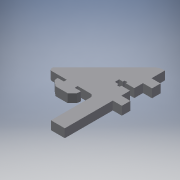
# Autodesk Inventor part: Y-Motor-Brace
Saved by Autodesk Inventor 2017 (Build 210142000, 142)
## iProperties
Created: 2016-07-21
Part Number: Y-Motor-Brace
Material: Generic
Document SubType Name: Modeling
Designer: User
Density: 1 g/cm^3
Appearance: Default
Author: User
Autodesk Inventor part; units mm, degrees
(part 1 of 2)
ref_plane "YZ Plane" through (0, 0, 0) normal (1, 0, 0) x (0, 1, 0)
ref_plane "XZ Plane" through (0, 0, 0) normal (0, 1, 0) x (-1, 0, 0)
ref_plane "XY Plane" through (0, 0, 0) normal (0, 0, 1) x (1, 0, 0)
sketch "Sketch1" plane through (0, 0, 0) normal (0, 0, 1) x (1, 0, 0)
  line L0 (977.8791, 108.9161) -> (977.8791, 115.0161)
  line L1 (977.8791, 115.0161) -> (984.2291, 115.0161)
  line L2 (984.2291, 115.0161) -> (984.2291, 121.0067)
  line L3 (984.2291, 121.0067) -> (977.8884, 121.0067)
  line L4 (977.8884, 121.0067) -> (977.8884, 130.4067)
  line L5 (977.8884, 130.4067) -> (977.2021, 130.4067)
  line L6 (977.2021, 130.4067) -> (976.6789, 130.3897)
  line L7 (976.6789, 130.3897) -> (976.1579, 130.3385)
  line L8 (976.1579, 130.3385) -> (975.6413, 130.2534)
  line L9 (975.6413, 130.2534) -> (975.1315, 130.1346)
  line L10 (975.1315, 130.1346) -> (974.6306, 129.9827)
  line L11 (974.6306, 129.9827) -> (974.1405, 129.7985)
  line L12 (974.1405, 129.7985) -> (973.6636, 129.5825)
  line L13 (973.6636, 129.5825) -> (973.2019, 129.3358)
  line L14 (973.2019, 129.3358) -> (972.7572, 129.0595)
  line L15 (972.7572, 129.0595) -> (972.3316, 128.7547)
  line L16 (972.3316, 128.7547) -> (971.9269, 128.4227)
  line L17 (971.9269, 128.4227) -> (971.5447, 128.0649)
  line L18 (971.5447, 128.0649) -> (937.996, 94.5327)
  line L19 (937.996, 94.5327) -> (938.0208, 94.542)
  line L20 (938.0208, 94.542) -> (937.2042, 93.7246)
  spline S0 degree 3 poles (937.2042, 93.7246) (937.0556, 93.5758) (936.9321, 93.4056) (936.8368, 93.2181) knots 21 21 21 21 22 22 22 22
  line L21 (937.2042, 93.7246) -> (937.0556, 93.5758) construction
  line L22 (937.0556, 93.5758) -> (936.9321, 93.4056) construction
  line L23 (936.9321, 93.4056) -> (936.8368, 93.2181) construction
  spline S1 degree 3 poles (936.8368, 93.2181) (936.7414, 93.0307) (936.6766, 92.8306) (936.6438, 92.6229) knots 22 22 22 22 23 23 23 23
  line L24 (936.8368, 93.2181) -> (936.7414, 93.0307) construction
  line L25 (936.7414, 93.0307) -> (936.6766, 92.8306) construction
  line L26 (936.6766, 92.8306) -> (936.6438, 92.6229) construction
  spline S2 degree 3 poles (936.6438, 92.6229) (936.611, 92.4151) (936.6112, 92.2048) (936.6443, 91.9971) (936.6774, 91.7895) (936.7425, 91.5895) (936.8381, 91.4022) knots 23 23 23 23 24 24 24 25 25 25 25
  line L27 (936.6438, 92.6229) -> (936.611, 92.4151) construction
  line L28 (936.611, 92.4151) -> (936.6112, 92.2048) construction
  line L29 (936.6112, 92.2048) -> (936.6443, 91.9971) construction
  line L30 (936.6443, 91.9971) -> (936.6774, 91.7895) construction
  line L31 (936.6774, 91.7895) -> (936.7425, 91.5895) construction
  line L32 (936.7425, 91.5895) -> (936.8381, 91.4022) construction
  spline S3 degree 3 poles (936.8381, 91.4022) (936.9337, 91.2148) (937.0574, 91.0448) (937.2062, 90.8962) knots 25 25 25 25 26 26 26 26
  line L33 (936.8381, 91.4022) -> (936.9337, 91.2148) construction
  line L34 (936.9337, 91.2148) -> (937.0574, 91.0448) construction
  line L35 (937.0574, 91.0448) -> (937.2062, 90.8962) construction
  spline S4 degree 3 poles (937.2062, 90.8962) (937.355, 90.7476) (937.5252, 90.6241) (937.7127, 90.5287) knots 26 26 26 26 27 27 27 27
  line L36 (937.2062, 90.8962) -> (937.355, 90.7476) construction
  line L37 (937.355, 90.7476) -> (937.5252, 90.6241) construction
  line L38 (937.5252, 90.6241) -> (937.7127, 90.5287) construction
  spline S5 degree 3 poles (937.7127, 90.5287) (937.9002, 90.4334) (938.1002, 90.3685) (938.3079, 90.3358) knots 27 27 27 27 28 28 28 28
  line L39 (937.7127, 90.5287) -> (937.9002, 90.4334) construction
  line L40 (937.9002, 90.4334) -> (938.1002, 90.3685) construction
  line L41 (938.1002, 90.3685) -> (938.3079, 90.3358) construction
  spline S6 degree 3 poles (938.3079, 90.3358) (938.411, 90.3195) (938.5151, 90.3114) (938.6195, 90.3114) knots 28 28 28 28 29 29 29 29
  line L42 (938.3079, 90.3358) -> (938.411, 90.3195) construction
  line L43 (938.411, 90.3195) -> (938.5151, 90.3114) construction
  line L44 (938.5151, 90.3114) -> (938.6195, 90.3114) construction
  line L45 (938.6195, 90.3114) -> (949.0602, 90.3114)
  line L46 (949.0602, 90.3114) -> (949.0602, 88.2628)
  line L47 (949.0602, 88.2628) -> (944.6963, 88.2628)
  line L48 (944.6963, 88.2628) -> (944.6963, 87.5628)
  line L49 (944.6963, 87.5628) -> (945.0555, 85.6914)
  line L50 (945.0555, 85.6914) -> (949.0203, 82.4161)
  line L51 (949.0203, 82.4161) -> (957.4678, 82.4161)
  line L52 (957.4678, 82.4161) -> (960.7553, 85.6883)
  line L53 (960.7553, 85.6883) -> (961.0631, 87.5612)
  line L54 (961.0631, 87.5612) -> (961.0631, 88.2612)
  line L55 (961.0631, 88.2612) -> (956.7022, 88.2612)
  line L56 (956.7022, 88.2612) -> (956.7022, 90.3082)
  line L57 (956.7022, 90.3082) -> (965.3221, 90.3082)
  line L58 (965.3221, 90.3082) -> (966.007, 90.2748)
  line L59 (966.007, 90.2748) -> (966.66, 90.0653)
  line L60 (966.66, 90.0653) -> (967.2366, 89.6939)
  line L61 (967.2366, 89.6939) -> (967.6973, 89.186)
  line L62 (967.6973, 89.186) -> (968.0109, 88.5761)
  line L63 (968.0109, 88.5761) -> (968.1559, 87.9058)
  line L64 (968.1559, 87.9058) -> (968.1559, 60.091)
  line L65 (968.1559, 60.091) -> (977.8791, 60.091)
  line L66 (977.8791, 60.091) -> (977.8791, 93.8161)
  line L67 (977.8791, 93.8161) -> (984.2291, 93.8161)
  line L68 (984.2291, 93.8161) -> (984.2291, 99.8161)
  line L69 (984.2291, 99.8161) -> (977.8791, 99.8161)
  line L70 (977.8791, 99.8161) -> (977.8791, 105.9161)
  line L71 (977.8791, 105.9161) -> (971.879, 105.9161)
  line L72 (971.879, 105.9161) -> (971.879, 104.6661)
  line L73 (971.879, 104.6661) -> (969.8791, 104.6661)
  line L74 (969.8791, 104.6661) -> (969.8791, 105.9161)
  line L75 (969.8791, 105.9161) -> (967.2291, 105.9161)
  line L76 (967.2291, 105.9161) -> (967.2291, 108.9161)
  line L77 (967.2291, 108.9161) -> (969.8791, 108.9161)
  line L78 (969.8791, 108.9161) -> (969.8791, 110.1661)
  line L79 (969.8791, 110.1661) -> (971.879, 110.1661)
  line L80 (971.879, 110.1661) -> (971.879, 108.9161)
  line L81 (971.879, 108.9161) -> (977.8791, 108.9161)
  line L82 (967.192, 195.3235) -> (966.942, 195.9235)
  line L83 (966.942, 195.9235) -> (966.542, 196.4485)
  line L84 (966.542, 196.4485) -> (966.017, 196.8485)
  line L85 (966.017, 196.8485) -> (965.417, 197.0985)
  line L86 (965.417, 197.0985) -> (964.767, 197.1985)
  line L87 (964.767, 197.1985) -> (964.117, 197.0984)
  line L88 (964.117, 197.0984) -> (963.492, 196.8484)
  line L89 (963.492, 196.8484) -> (962.967, 196.4484)
  line L90 (962.967, 196.4484) -> (962.567, 195.9234)
  line L91 (962.567, 195.9234) -> (962.317, 195.3234)
  line L92 (962.317, 195.3234) -> (962.242, 194.6734)
  line L93 (962.242, 194.6734) -> (962.3171, 194.0234)
  line L94 (962.3171, 194.0234) -> (962.5671, 193.3984)
  line L95 (962.5671, 193.3984) -> (962.9671, 192.8984)
  line L96 (962.9671, 192.8984) -> (963.492, 192.4985)
  line L97 (963.492, 192.4985) -> (964.1171, 192.2485)
  line L98 (964.1171, 192.2485) -> (964.7671, 192.1486)
  line L99 (964.7671, 192.1486) -> (965.4171, 192.2486)
  line L100 (965.4171, 192.2486) -> (966.017, 192.4987)
  line L101 (966.017, 192.4987) -> (966.5421, 192.8987)
  line L102 (966.5421, 192.8987) -> (966.9422, 193.3986)
  line L103 (966.9422, 193.3986) -> (967.1921, 194.0236)
  line L104 (967.1921, 194.0236) -> (967.2671, 194.6733)
  line L105 (967.2671, 194.6733) -> (967.192, 195.3235)
  line L106 (983.267, 191.6734) -> (983.267, 185.2734)
  line L107 (983.267, 185.2734) -> (989.467, 185.2734)
  line L108 (989.467, 185.2734) -> (989.467, 191.6734)
  line L109 (989.467, 191.6734) -> (983.267, 191.6734)
  line L110 (987.3418, 197.698) -> (987.3418, 197.798)
  line L111 (987.3418, 197.798) -> (987.3169, 197.898)
  line L112 (987.3169, 197.898) -> (987.2669, 197.998)
  line L113 (987.2669, 197.998) -> (987.2419, 198.098)
  line L114 (987.2419, 198.098) -> (987.1919, 198.198)
  line L115 (987.1919, 198.198) -> (987.1419, 198.298)
  line L116 (987.1419, 198.298) -> (987.0919, 198.373)
  line L117 (987.0919, 198.373) -> (987.042, 198.473)
  line L118 (987.042, 198.473) -> (986.9669, 198.548)
  line L119 (986.9669, 198.548) -> (986.892, 198.6231)
  line L120 (986.892, 198.6231) -> (986.817, 198.6981)
  line L121 (986.817, 198.6981) -> (986.742, 198.7481)
  line L122 (986.742, 198.7481) -> (986.642, 198.8231)
  line L123 (986.642, 198.8231) -> (986.567, 198.8731)
  line L124 (986.567, 198.8731) -> (986.467, 198.9232)
  line L125 (986.467, 198.9232) -> (986.3671, 198.9732)
  line L126 (986.3671, 198.9732) -> (986.2671, 198.9983)
  line L127 (986.2671, 198.9983) -> (986.1671, 199.0483)
  line L128 (986.1671, 199.0483) -> (986.0671, 199.0483)
  line L129 (986.0671, 199.0483) -> (985.9671, 199.0734)
  line L130 (985.9671, 199.0734) -> (985.8671, 199.0983)
  line L131 (985.8671, 199.0983) -> (985.7671, 199.0983)
  line L132 (985.7671, 199.0983) -> (985.6671, 199.0983)
  line L133 (985.6671, 199.0983) -> (985.5422, 199.0734)
  line L134 (985.5422, 199.0734) -> (985.4421, 199.0483)
  line L135 (985.4421, 199.0483) -> (985.3421, 199.0483)
  line L136 (985.3421, 199.0483) -> (985.2421, 198.9983)
  line L137 (985.2421, 198.9983) -> (985.1421, 198.9733)
  line L138 (985.1421, 198.9733) -> (985.0421, 198.9234)
  line L139 (985.0421, 198.9234) -> (984.9671, 198.8733)
  line L140 (984.9671, 198.8733) -> (984.8671, 198.8234)
  line L141 (984.8671, 198.8234) -> (984.7922, 198.7484)
  line L142 (984.7922, 198.7484) -> (984.7171, 198.6984)
  line L143 (984.7171, 198.6984) -> (984.6421, 198.6234)
  line L144 (984.6421, 198.6234) -> (984.5671, 198.5484)
  line L145 (984.5671, 198.5484) -> (984.4921, 198.4734)
  line L146 (984.4921, 198.4734) -> (984.4421, 198.3734)
  line L147 (984.4421, 198.3734) -> (984.3671, 198.2984)
  line L148 (984.3671, 198.2984) -> (984.317, 198.1984)
  line L149 (984.317, 198.1984) -> (984.292, 198.0984)
  line L150 (984.292, 198.0984) -> (984.2421, 197.9984)
  line L151 (984.2421, 197.9984) -> (984.2171, 197.8985)
  line L152 (984.2171, 197.8985) -> (984.192, 197.7984)
  line L153 (984.192, 197.7984) -> (984.167, 197.6984)
  line L154 (984.167, 197.6984) -> (984.167, 197.5984)
  line L155 (984.167, 197.5984) -> (984.167, 197.4984)
  line L156 (984.167, 197.4984) -> (984.167, 197.3984)
  line L157 (984.167, 197.3984) -> (984.167, 197.2734)
  line L158 (984.167, 197.2734) -> (984.192, 197.1734)
  line L159 (984.192, 197.1734) -> (984.2171, 197.0734)
  line L160 (984.2171, 197.0734) -> (984.2421, 196.9734)
  line L161 (984.2421, 196.9734) -> (984.2921, 196.8734)
  line L162 (984.2921, 196.8734) -> (984.317, 196.7734)
  line L163 (984.317, 196.7734) -> (984.3671, 196.6985)
  line L164 (984.3671, 196.6985) -> (984.4421, 196.5985)
  line L165 (984.4421, 196.5985) -> (984.4921, 196.5235)
  line L166 (984.4921, 196.5235) -> (984.5671, 196.4235)
  line L167 (984.5671, 196.4235) -> (984.6421, 196.3485)
  line L168 (984.6421, 196.3485) -> (984.7171, 196.2984)
  line L169 (984.7171, 196.2984) -> (984.7921, 196.2234)
  line L170 (984.7921, 196.2234) -> (984.867, 196.1484)
  line L171 (984.867, 196.1484) -> (984.967, 196.0983)
  line L172 (984.967, 196.0983) -> (985.042, 196.0483)
  line L173 (985.042, 196.0483) -> (985.142, 196.0233)
  line L174 (985.142, 196.0233) -> (985.2419, 195.9732)
  line L175 (985.2419, 195.9732) -> (985.3419, 195.9482)
  line L176 (985.3419, 195.9482) -> (985.4419, 195.9231)
  line L177 (985.4419, 195.9231) -> (985.542, 195.8981)
  line L178 (985.542, 195.8981) -> (985.6669, 195.8981)
  line L179 (985.6669, 195.8981) -> (985.7669, 195.8981)
  line L180 (985.7669, 195.8981) -> (985.8669, 195.8981)
  line L181 (985.8669, 195.8981) -> (985.9669, 195.8981)
  line L182 (985.9669, 195.8981) -> (986.0669, 195.9231)
  line L183 (986.0669, 195.9231) -> (986.1669, 195.9481)
  line L184 (986.1669, 195.9481) -> (986.2669, 195.9731)
  line L185 (986.2669, 195.9731) -> (986.3669, 196.0231)
  line L186 (986.3669, 196.0231) -> (986.4669, 196.0482)
  line L187 (986.4669, 196.0482) -> (986.5669, 196.0981)
  line L188 (986.5669, 196.0981) -> (986.6419, 196.1481)
  line L189 (986.6419, 196.1481) -> (986.7419, 196.2231)
  line L190 (986.7419, 196.2231) -> (986.8169, 196.2981)
  line L191 (986.8169, 196.2981) -> (986.8919, 196.3481)
  line L192 (986.8919, 196.3481) -> (986.9669, 196.4231)
  line L193 (986.9669, 196.4231) -> (987.042, 196.5231)
  line L194 (987.042, 196.5231) -> (987.092, 196.5981)
  line L195 (987.092, 196.5981) -> (987.1419, 196.6981)
  line L196 (987.1419, 196.6981) -> (987.192, 196.7731)
  line L197 (987.192, 196.7731) -> (987.242, 196.8731)
  line L198 (987.242, 196.8731) -> (987.267, 196.9731)
  line L199 (987.267, 196.9731) -> (987.3169, 197.0731)
  line L200 (987.3169, 197.0731) -> (987.3419, 197.1731)
  line L201 (987.3419, 197.1731) -> (987.3419, 197.2731)
  line L202 (987.3419, 197.2731) -> (987.3669, 197.398)
  line L203 (987.3669, 197.398) -> (987.3669, 197.4979)
  line L204 (987.3669, 197.4979) -> (987.3669, 197.598)
  line L205 (987.3669, 197.598) -> (987.3418, 197.698)
  line L206 (1012.7431, 213.7485) -> (1012.6681, 214.4985)
  line L207 (1012.6681, 214.4985) -> (1012.5425, 215.2239)
  line L208 (1012.5425, 215.2239) -> (1012.3674, 215.9738)
  line L209 (1012.3674, 215.9738) -> (1012.1423, 216.6988)
  line L210 (1012.1423, 216.6988) -> (1011.8923, 217.3988)
  line L211 (1011.8923, 217.3988) -> (1011.5673, 218.0738)
  line L212 (1011.5673, 218.0738) -> (1011.2173, 218.7488)
  line L213 (1011.2173, 218.7488) -> (1010.8173, 219.3738)
  line L214 (1010.8173, 219.3738) -> (1010.3922, 219.9987)
  line L215 (1010.3922, 219.9987) -> (1009.917, 220.5735)
  line L216 (1009.917, 220.5735) -> (1009.3919, 221.1234)
  line L217 (1009.3919, 221.1234) -> (1008.8419, 221.6485)
  line L218 (1008.8419, 221.6485) -> (1008.2669, 222.1234)
  line L219 (1008.2669, 222.1234) -> (1007.6419, 222.5484)
  line L220 (1007.6419, 222.5484) -> (1007.0169, 222.9484)
  line L221 (1007.0169, 222.9484) -> (1006.3419, 223.2984)
  line L222 (1006.3419, 223.2984) -> (1005.6669, 223.6234)
  line L223 (1005.6669, 223.6234) -> (1004.967, 223.8735)
  line L224 (1004.967, 223.8735) -> (1004.2419, 224.0985)
  line L225 (1004.2419, 224.0985) -> (1003.5169, 224.2736)
  line L226 (1003.5169, 224.2736) -> (1002.7669, 224.3986)
  line L227 (1002.7669, 224.3986) -> (1002.017, 224.4737)
  line L228 (1002.017, 224.4737) -> (1001.267, 224.4987)
  line L229 (1001.267, 224.4987) -> (1000.517, 224.4737)
  line L230 (1000.517, 224.4737) -> (999.767, 224.3986)
  line L231 (999.767, 224.3986) -> (999.017, 224.2737)
  line L232 (999.017, 224.2737) -> (998.2919, 224.0987)
  line L233 (998.2919, 224.0987) -> (997.5669, 223.8736)
  line L234 (997.5669, 223.8736) -> (996.8669, 223.6236)
  line L235 (996.8669, 223.6236) -> (996.1669, 223.2986)
  line L236 (996.1669, 223.2986) -> (995.5169, 222.9486)
  line L237 (995.5169, 222.9486) -> (994.8669, 222.5486)
  line L238 (994.8669, 222.5486) -> (994.2671, 222.1234)
  line L239 (994.2671, 222.1234) -> (993.6672, 221.6483)
  line L240 (993.6672, 221.6483) -> (993.142, 221.1234)
  line L241 (993.142, 221.1234) -> (992.617, 220.5734)
  line L242 (992.617, 220.5734) -> (992.142, 219.9984)
  line L243 (992.142, 219.9984) -> (991.692, 219.3735)
  line L244 (991.692, 219.3735) -> (991.292, 218.7484)
  line L245 (991.292, 218.7484) -> (990.942, 218.0734)
  line L246 (990.942, 218.0734) -> (990.642, 217.3984)
  line L247 (990.642, 217.3984) -> (990.367, 216.6984)
  line L248 (990.367, 216.6984) -> (990.142, 215.9734)
  line L249 (990.142, 215.9734) -> (989.992, 215.2234)
  line L250 (989.992, 215.2234) -> (989.8671, 214.4984)
  line L251 (989.8671, 214.4984) -> (989.792, 213.7484)
  line L252 (989.792, 213.7484) -> (989.767, 212.9984)
  line L253 (989.767, 212.9984) -> (989.792, 212.2484)
  line L254 (989.792, 212.2484) -> (989.8671, 211.4984)
  line L255 (989.8671, 211.4984) -> (989.992, 210.7484)
  line L256 (989.992, 210.7484) -> (990.142, 210.0234)
  line L257 (990.142, 210.0234) -> (990.367, 209.2984)
  line L258 (990.367, 209.2984) -> (990.642, 208.5984)
  line L259 (990.642, 208.5984) -> (990.942, 207.8984)
  line L260 (990.942, 207.8984) -> (991.292, 207.2484)
  line L261 (991.292, 207.2484) -> (991.692, 206.5984)
  line L262 (991.692, 206.5984) -> (992.1421, 205.9985)
  line L263 (992.1421, 205.9985) -> (992.6172, 205.3986)
  line L264 (992.6172, 205.3986) -> (993.1424, 204.8487)
  line L265 (993.1424, 204.8487) -> (993.6674, 204.3488)
  line L266 (993.6674, 204.3488) -> (994.2675, 203.8739)
  line L267 (994.2675, 203.8739) -> (994.8673, 203.4237)
  line L268 (994.8673, 203.4237) -> (995.5172, 203.0235)
  line L269 (995.5172, 203.0235) -> (996.1671, 202.6732)
  line L270 (996.1671, 202.6732) -> (996.8669, 202.373)
  line L271 (996.8669, 202.373) -> (997.567, 202.098)
  line L272 (997.567, 202.098) -> (998.292, 201.8729)
  line L273 (998.292, 201.8729) -> (999.017, 201.7229)
  line L274 (999.017, 201.7229) -> (999.767, 201.5978)
  line L275 (999.767, 201.5978) -> (1000.517, 201.5228)
  line L276 (1000.517, 201.5228) -> (1001.267, 201.4978)
  line L277 (1001.267, 201.4978) -> (1002.017, 201.5228)
  line L278 (1002.017, 201.5228) -> (1002.767, 201.5978)
  line L279 (1002.767, 201.5978) -> (1003.517, 201.7228)
  line L280 (1003.517, 201.7228) -> (1004.242, 201.8727)
  line L281 (1004.242, 201.8727) -> (1004.967, 202.0978)
  line L282 (1004.967, 202.0978) -> (1005.6669, 202.3728)
  line L283 (1005.6669, 202.3728) -> (1006.3419, 202.6728)
  line L284 (1006.3419, 202.6728) -> (1007.017, 203.0228)
  line L285 (1007.017, 203.0228) -> (1007.6419, 203.4228)
  line L286 (1007.6419, 203.4228) -> (1008.2669, 203.8728)
  line L287 (1008.2669, 203.8728) -> (1008.8419, 204.3478)
  line L288 (1008.8419, 204.3478) -> (1009.3919, 204.8478)
  line L289 (1009.3919, 204.8478) -> (1009.9169, 205.3978)
  line L290 (1009.9169, 205.3978) -> (1010.3921, 205.9977)
  line L291 (1010.3921, 205.9977) -> (1010.8171, 206.5977)
  line L292 (1010.8171, 206.5977) -> (1011.2173, 207.2475)
  line L293 (1011.2173, 207.2475) -> (1011.5675, 207.8974)
  line L294 (1011.5675, 207.8974) -> (1011.8928, 208.5973)
  line L295 (1011.8928, 208.5973) -> (1012.1428, 209.2973)
  line L296 (1012.1428, 209.2973) -> (1012.3679, 210.0223)
  line L297 (1012.3679, 210.0223) -> (1012.5429, 210.7473)
  line L298 (1012.5429, 210.7473) -> (1012.6679, 211.4973)
  line L299 (1012.6679, 211.4973) -> (1012.743, 212.2473)
  line L300 (1012.743, 212.2473) -> (1012.7681, 212.9999)
  line L301 (1012.7681, 212.9999) -> (1012.7431, 213.7485)
  line L302 (998.542, 188.6729) -> (998.542, 188.7729)
  line L303 (998.542, 188.7729) -> (998.5169, 188.8729)
  line L304 (998.5169, 188.8729) -> (998.467, 188.9729)
  line L305 (998.467, 188.9729) -> (998.442, 189.0729)
  line L306 (998.442, 189.0729) -> (998.392, 189.1729)
  line L307 (998.392, 189.1729) -> (998.342, 189.2729)
  line L308 (998.342, 189.2729) -> (998.292, 189.3479)
  line L309 (998.292, 189.3479) -> (998.242, 189.4479)
  line L310 (998.242, 189.4479) -> (998.167, 189.523)
  line L311 (998.167, 189.523) -> (998.092, 189.598)
  line L312 (998.092, 189.598) -> (998.0171, 189.673)
  line L313 (998.0171, 189.673) -> (997.9421, 189.748)
  line L314 (997.9421, 189.748) -> (997.8421, 189.7981)
  line L315 (997.8421, 189.7981) -> (997.7671, 189.8481)
  line L316 (997.7671, 189.8481) -> (997.6671, 189.8982)
  line L317 (997.6671, 189.8982) -> (997.5671, 189.9482)
  line L318 (997.5671, 189.9482) -> (997.4672, 189.9732)
  line L319 (997.4672, 189.9732) -> (997.3672, 190.0233)
  line L320 (997.3672, 190.0233) -> (997.2672, 190.0483)
  line L321 (997.2672, 190.0483) -> (997.1672, 190.0483)
  line L322 (997.1672, 190.0483) -> (997.0672, 190.0734)
  line L323 (997.0672, 190.0734) -> (996.9672, 190.0734)
  line L324 (996.9672, 190.0734) -> (996.8671, 190.0734)
  line L325 (996.8671, 190.0734) -> (996.7422, 190.0483)
  line L326 (996.7422, 190.0483) -> (996.6421, 190.0483)
  line L327 (996.6421, 190.0483) -> (996.5422, 190.0233)
  line L328 (996.5422, 190.0233) -> (996.4421, 189.9733)
  line L329 (996.4421, 189.9733) -> (996.3421, 189.9483)
  line L330 (996.3421, 189.9483) -> (996.2421, 189.8984)
  line L331 (996.2421, 189.8984) -> (996.1671, 189.8484)
  line L332 (996.1671, 189.8484) -> (996.0671, 189.7984)
  line L333 (996.0671, 189.7984) -> (995.9921, 189.7484)
  line L334 (995.9921, 189.7484) -> (995.9171, 189.6734)
  line L335 (995.9171, 189.6734) -> (995.8421, 189.5984)
  line L336 (995.8421, 189.5984) -> (995.7671, 189.5234)
  line L337 (995.7671, 189.5234) -> (995.6921, 189.4484)
  line L338 (995.6921, 189.4484) -> (995.6421, 189.3484)
  line L339 (995.6421, 189.3484) -> (995.5671, 189.2734)
  line L340 (995.5671, 189.2734) -> (995.5171, 189.1734)
  line L341 (995.5171, 189.1734) -> (995.4921, 189.0734)
  line L342 (995.4921, 189.0734) -> (995.4421, 188.9734)
  line L343 (995.4421, 188.9734) -> (995.417, 188.8734)
  line L344 (995.417, 188.8734) -> (995.3921, 188.7734)
  line L345 (995.3921, 188.7734) -> (995.3671, 188.6734)
  line L346 (995.3671, 188.6734) -> (995.3671, 188.5734)
  line L347 (995.3671, 188.5734) -> (995.3671, 188.4734)
  line L348 (995.3671, 188.4734) -> (995.3671, 188.3735)
  line L349 (995.3671, 188.3735) -> (995.3671, 188.2734)
  line L350 (995.3671, 188.2734) -> (995.392, 188.1484)
  line L351 (995.392, 188.1484) -> (995.417, 188.0484)
  line L352 (995.417, 188.0484) -> (995.4421, 187.9484)
  line L353 (995.4421, 187.9484) -> (995.4921, 187.8484)
  line L354 (995.4921, 187.8484) -> (995.517, 187.7735)
  line L355 (995.517, 187.7735) -> (995.5671, 187.6734)
  line L356 (995.5671, 187.6734) -> (995.6421, 187.5734)
  line L357 (995.6421, 187.5734) -> (995.6921, 187.4984)
  line L358 (995.6921, 187.4984) -> (995.767, 187.4234)
  line L359 (995.767, 187.4234) -> (995.842, 187.3484)
  line L360 (995.842, 187.3484) -> (995.9169, 187.2733)
  line L361 (995.9169, 187.2733) -> (995.9919, 187.1983)
  line L362 (995.9919, 187.1983) -> (996.0669, 187.1483)
  line L363 (996.0669, 187.1483) -> (996.1669, 187.0733)
  line L364 (996.1669, 187.0733) -> (996.2419, 187.0233)
  line L365 (996.2419, 187.0233) -> (996.3419, 186.9982)
  line L366 (996.3419, 186.9982) -> (996.4418, 186.9482)
  line L367 (996.4418, 186.9482) -> (996.5419, 186.9232)
  line L368 (996.5419, 186.9232) -> (996.6418, 186.8981)
  line L369 (996.6418, 186.8981) -> (996.7419, 186.8731)
  line L370 (996.7419, 186.8731) -> (996.8668, 186.8731)
  line L371 (996.8668, 186.8731) -> (996.9669, 186.8731)
  line L372 (996.9669, 186.8731) -> (997.0669, 186.8731)
  line L373 (997.0669, 186.8731) -> (997.1668, 186.8731)
  line L374 (997.1668, 186.8731) -> (997.2668, 186.8981)
  line L375 (997.2668, 186.8981) -> (997.3668, 186.9231)
  line L376 (997.3668, 186.9231) -> (997.4668, 186.9481)
  line L377 (997.4668, 186.9481) -> (997.5668, 186.9981)
  line L378 (997.5668, 186.9981) -> (997.6668, 187.0231)
  line L379 (997.6668, 187.0231) -> (997.7668, 187.0731)
  line L380 (997.7668, 187.0731) -> (997.8418, 187.1481)
  line L381 (997.8418, 187.1481) -> (997.9418, 187.198)
  line L382 (997.9418, 187.198) -> (998.0169, 187.273)
  line L383 (998.0169, 187.273) -> (998.0919, 187.348)
  line L384 (998.0919, 187.348) -> (998.1669, 187.423)
  line L385 (998.1669, 187.423) -> (998.242, 187.498)
  line L386 (998.242, 187.498) -> (998.2919, 187.573)
  line L387 (998.2919, 187.573) -> (998.3419, 187.673)
  line L388 (998.3419, 187.673) -> (998.392, 187.773)
  line L389 (998.392, 187.773) -> (998.442, 187.848)
  line L390 (998.442, 187.848) -> (998.467, 187.948)
  line L391 (998.467, 187.948) -> (998.5169, 188.048)
  line L392 (998.5169, 188.048) -> (998.542, 188.148)
  line L393 (998.542, 188.148) -> (998.542, 188.273)
  line L394 (998.542, 188.273) -> (998.567, 188.373)
  line L395 (998.567, 188.373) -> (998.567, 188.473)
  line L396 (998.567, 188.473) -> (998.567, 188.5729)
  line L397 (998.567, 188.5729) -> (998.542, 188.6729)
  line L398 (1004.467, 191.6734) -> (1004.467, 185.2734)
  line L399 (1004.467, 185.2734) -> (1010.667, 185.2734)
  line L400 (1010.667, 185.2734) -> (1010.667, 191.6734)
  line L401 (1010.667, 191.6734) -> (1004.467, 191.6734)
  line L402 (1018.3418, 197.698) -> (1018.3418, 197.798)
  line L403 (1018.3418, 197.798) -> (1018.3168, 197.8981)
  line L404 (1018.3168, 197.8981) -> (1018.2669, 197.998)
  line L405 (1018.2669, 197.998) -> (1018.2419, 198.098)
  line L406 (1018.2419, 198.098) -> (1018.1919, 198.198)
  line L407 (1018.1919, 198.198) -> (1018.1418, 198.2981)
  line L408 (1018.1418, 198.2981) -> (1018.0919, 198.373)
  line L409 (1018.0919, 198.373) -> (1018.0419, 198.4731)
  line L410 (1018.0419, 198.4731) -> (1017.9669, 198.5481)
  line L411 (1017.9669, 198.5481) -> (1017.892, 198.6231)
  line L412 (1017.892, 198.6231) -> (1017.817, 198.6981)
  line L413 (1017.817, 198.6981) -> (1017.742, 198.7482)
  line L414 (1017.742, 198.7482) -> (1017.642, 198.8232)
  line L415 (1017.642, 198.8232) -> (1017.567, 198.8732)
  line L416 (1017.567, 198.8732) -> (1017.467, 198.9233)
  line L417 (1017.467, 198.9233) -> (1017.367, 198.9733)
  line L418 (1017.367, 198.9733) -> (1017.2671, 198.9983)
  line L419 (1017.2671, 198.9983) -> (1017.1671, 199.0484)
  line L420 (1017.1671, 199.0484) -> (1017.0671, 199.0484)
  line L421 (1017.0671, 199.0484) -> (1016.9671, 199.0734)
  line L422 (1016.9671, 199.0734) -> (1016.8671, 199.0984)
  line L423 (1016.8671, 199.0984) -> (1016.7671, 199.0984)
  line L424 (1016.7671, 199.0984) -> (1016.6671, 199.0984)
  line L425 (1016.6671, 199.0984) -> (1016.5422, 199.0734)
  line L426 (1016.5422, 199.0734) -> (1016.4421, 199.0484)
  line L427 (1016.4421, 199.0484) -> (1016.3421, 199.0484)
  line L428 (1016.3421, 199.0484) -> (1016.2421, 198.9984)
  line L429 (1016.2421, 198.9984) -> (1016.1421, 198.9734)
  line L430 (1016.1421, 198.9734) -> (1016.0421, 198.9234)
  line L431 (1016.0421, 198.9234) -> (1015.9672, 198.8734)
  line L432 (1015.9672, 198.8734) -> (1015.8671, 198.8234)
  line L433 (1015.8671, 198.8234) -> (1015.7922, 198.7484)
  line L434 (1015.7922, 198.7484) -> (1015.7171, 198.6984)
  line L435 (1015.7171, 198.6984) -> (1015.6422, 198.6234)
  line L436 (1015.6422, 198.6234) -> (1015.5671, 198.5484)
  line L437 (1015.5671, 198.5484) -> (1015.4921, 198.4734)
  line L438 (1015.4921, 198.4734) -> (1015.4421, 198.3734)
  line L439 (1015.4421, 198.3734) -> (1015.3671, 198.2984)
  line L440 (1015.3671, 198.2984) -> (1015.317, 198.1984)
  line L441 (1015.317, 198.1984) -> (1015.2921, 198.0984)
  line L442 (1015.2921, 198.0984) -> (1015.242, 197.9984)
  line L443 (1015.242, 197.9984) -> (1015.217, 197.8984)
  line L444 (1015.217, 197.8984) -> (1015.192, 197.7984)
  line L445 (1015.192, 197.7984) -> (1015.167, 197.6984)
  line L446 (1015.167, 197.6984) -> (1015.167, 197.5984)
  line L447 (1015.167, 197.5984) -> (1015.167, 197.4984)
  line L448 (1015.167, 197.4984) -> (1015.167, 197.3984)
  line L449 (1015.167, 197.3984) -> (1015.167, 197.2734)
  line L450 (1015.167, 197.2734) -> (1015.192, 197.1734)
  line L451 (1015.192, 197.1734) -> (1015.217, 197.0734)
  line L452 (1015.217, 197.0734) -> (1015.242, 196.9734)
  line L453 (1015.242, 196.9734) -> (1015.292, 196.8734)
  line L454 (1015.292, 196.8734) -> (1015.317, 196.7734)
  line L455 (1015.317, 196.7734) -> (1015.3671, 196.6984)
  line L456 (1015.3671, 196.6984) -> (1015.4421, 196.5984)
  line L457 (1015.4421, 196.5984) -> (1015.4921, 196.5234)
  line L458 (1015.4921, 196.5234) -> (1015.5671, 196.4235)
  line L459 (1015.5671, 196.4235) -> (1015.6421, 196.3485)
  line L460 (1015.6421, 196.3485) -> (1015.717, 196.2984)
  line L461 (1015.717, 196.2984) -> (1015.7921, 196.2234)
  line L462 (1015.7921, 196.2234) -> (1015.867, 196.1484)
  line L463 (1015.867, 196.1484) -> (1015.9671, 196.0984)
  line L464 (1015.9671, 196.0984) -> (1016.042, 196.0484)
  line L465 (1016.042, 196.0484) -> (1016.142, 196.0233)
  line L466 (1016.142, 196.0233) -> (1016.2419, 195.9733)
  line L467 (1016.2419, 195.9733) -> (1016.3419, 195.9482)
  line L468 (1016.3419, 195.9482) -> (1016.4419, 195.9232)
  line L469 (1016.4419, 195.9232) -> (1016.542, 195.8982)
  line L470 (1016.542, 195.8982) -> (1016.667, 195.8982)
  line L471 (1016.667, 195.8982) -> (1016.7669, 195.8982)
  line L472 (1016.7669, 195.8982) -> (1016.8669, 195.8982)
  line L473 (1016.8669, 195.8982) -> (1016.9669, 195.8982)
  line L474 (1016.9669, 195.8982) -> (1017.0669, 195.9231)
  line L475 (1017.0669, 195.9231) -> (1017.1669, 195.9482)
  line L476 (1017.1669, 195.9482) -> (1017.2669, 195.9732)
  line L477 (1017.2669, 195.9732) -> (1017.3669, 196.0232)
  line L478 (1017.3669, 196.0232) -> (1017.4669, 196.0482)
  line L479 (1017.4669, 196.0482) -> (1017.5669, 196.0982)
  line L480 (1017.5669, 196.0982) -> (1017.6419, 196.1481)
  line L481 (1017.6419, 196.1481) -> (1017.7419, 196.2232)
  line L482 (1017.7419, 196.2232) -> (1017.8169, 196.2981)
  line L483 (1017.8169, 196.2981) -> (1017.892, 196.3482)
  line L484 (1017.892, 196.3482) -> (1017.9669, 196.4232)
  line L485 (1017.9669, 196.4232) -> (1018.0419, 196.5231)
  line L486 (1018.0419, 196.5231) -> (1018.0919, 196.5981)
  line L487 (1018.0919, 196.5981) -> (1018.1419, 196.6982)
  line L488 (1018.1419, 196.6982) -> (1018.1919, 196.7731)
  line L489 (1018.1919, 196.7731) -> (1018.242, 196.8731)
  line L490 (1018.242, 196.8731) -> (1018.267, 196.9731)
  line L491 (1018.267, 196.9731) -> (1018.3169, 197.0731)
  line L492 (1018.3169, 197.0731) -> (1018.3419, 197.1731)
  line L493 (1018.3419, 197.1731) -> (1018.3419, 197.2731)
  line L494 (1018.3419, 197.2731) -> (1018.3669, 197.3981)
  line L495 (1018.3669, 197.3981) -> (1018.3669, 197.498)
  line L496 (1018.3669, 197.498) -> (1018.3669, 197.5981)
  line L497 (1018.3669, 197.5981) -> (1018.3418, 197.698)
  line L498 (1018.3419, 228.698) -> (1018.3419, 228.798)
  line L499 (1018.3419, 228.798) -> (1018.3169, 228.898)
  line L500 (1018.3169, 228.898) -> (1018.2669, 228.998)
  line L501 (1018.2669, 228.998) -> (1018.2419, 229.098)
  line L502 (1018.2419, 229.098) -> (1018.1919, 229.198)
  line L503 (1018.1919, 229.198) -> (1018.1419, 229.298)
  line L504 (1018.1419, 229.298) -> (1018.0919, 229.373)
  line L505 (1018.0919, 229.373) -> (1018.0419, 229.473)
  line L506 (1018.0419, 229.473) -> (1017.9669, 229.548)
  line L507 (1017.9669, 229.548) -> (1017.892, 229.623)
  line L508 (1017.892, 229.623) -> (1017.817, 229.6981)
  line L509 (1017.817, 229.6981) -> (1017.742, 229.7481)
  line L510 (1017.742, 229.7481) -> (1017.6421, 229.8231)
  line L511 (1017.6421, 229.8231) -> (1017.5671, 229.8731)
  line L512 (1017.5671, 229.8731) -> (1017.4671, 229.9232)
  line L513 (1017.4671, 229.9232) -> (1017.3671, 229.9732)
  line L514 (1017.3671, 229.9732) -> (1017.2671, 229.9983)
  line L515 (1017.2671, 229.9983) -> (1017.1671, 230.0483)
  line L516 (1017.1671, 230.0483) -> (1017.0672, 230.0483)
  line L517 (1017.0672, 230.0483) -> (1016.9672, 230.0734)
  line L518 (1016.9672, 230.0734) -> (1016.8672, 230.0983)
  line L519 (1016.8672, 230.0983) -> (1016.7672, 230.0983)
  line L520 (1016.7672, 230.0983) -> (1016.6672, 230.0983)
  line L521 (1016.6672, 230.0983) -> (1016.5422, 230.0734)
  line L522 (1016.5422, 230.0734) -> (1016.4421, 230.0483)
  line L523 (1016.4421, 230.0483) -> (1016.3421, 230.0483)
  line L524 (1016.3421, 230.0483) -> (1016.2421, 229.9984)
  line L525 (1016.2421, 229.9984) -> (1016.1421, 229.9734)
  line L526 (1016.1421, 229.9734) -> (1016.0422, 229.9234)
  line L527 (1016.0422, 229.9234) -> (1015.9672, 229.8733)
  line L528 (1015.9672, 229.8733) -> (1015.8671, 229.8233)
  line L529 (1015.8671, 229.8233) -> (1015.7922, 229.7483)
  line L530 (1015.7922, 229.7483) -> (1015.7171, 229.6984)
  line L531 (1015.7171, 229.6984) -> (1015.6421, 229.6234)
  line L532 (1015.6421, 229.6234) -> (1015.5671, 229.5484)
  line L533 (1015.5671, 229.5484) -> (1015.4921, 229.4734)
  line L534 (1015.4921, 229.4734) -> (1015.4421, 229.3734)
  line L535 (1015.4421, 229.3734) -> (1015.3671, 229.2984)
  line L536 (1015.3671, 229.2984) -> (1015.3171, 229.1984)
  line L537 (1015.3171, 229.1984) -> (1015.2921, 229.0984)
  line L538 (1015.2921, 229.0984) -> (1015.242, 228.9984)
  line L539 (1015.242, 228.9984) -> (1015.217, 228.8985)
  line L540 (1015.217, 228.8985) -> (1015.192, 228.7984)
  line L541 (1015.192, 228.7984) -> (1015.167, 228.6984)
  line L542 (1015.167, 228.6984) -> (1015.167, 228.5984)
  line L543 (1015.167, 228.5984) -> (1015.167, 228.4984)
  line L544 (1015.167, 228.4984) -> (1015.167, 228.3984)
  line L545 (1015.167, 228.3984) -> (1015.167, 228.2734)
  line L546 (1015.167, 228.2734) -> (1015.192, 228.1735)
  line L547 (1015.192, 228.1735) -> (1015.217, 228.0734)
  line L548 (1015.217, 228.0734) -> (1015.242, 227.9734)
  line L549 (1015.242, 227.9734) -> (1015.292, 227.8734)
  line L550 (1015.292, 227.8734) -> (1015.317, 227.7734)
  line L551 (1015.317, 227.7734) -> (1015.3671, 227.6984)
  line L552 (1015.3671, 227.6984) -> (1015.4421, 227.5984)
  line L553 (1015.4421, 227.5984) -> (1015.4921, 227.5235)
  line L554 (1015.4921, 227.5235) -> (1015.5671, 227.4235)
  line L555 (1015.5671, 227.4235) -> (1015.6421, 227.3484)
  line L556 (1015.6421, 227.3484) -> (1015.717, 227.2984)
  line L557 (1015.717, 227.2984) -> (1015.7921, 227.2234)
  line L558 (1015.7921, 227.2234) -> (1015.867, 227.1483)
  line L559 (1015.867, 227.1483) -> (1015.9671, 227.0984)
  line L560 (1015.9671, 227.0984) -> (1016.042, 227.0484)
  line L561 (1016.042, 227.0484) -> (1016.142, 227.0233)
  line L562 (1016.142, 227.0233) -> (1016.242, 226.9733)
  line L563 (1016.242, 226.9733) -> (1016.3419, 226.9482)
  line L564 (1016.3419, 226.9482) -> (1016.4419, 226.9232)
  line L565 (1016.4419, 226.9232) -> (1016.542, 226.8982)
  line L566 (1016.542, 226.8982) -> (1016.667, 226.8982)
  line L567 (1016.667, 226.8982) -> (1016.767, 226.8982)
  line L568 (1016.767, 226.8982) -> (1016.867, 226.8982)
  line L569 (1016.867, 226.8982) -> (1016.9669, 226.8982)
  line L570 (1016.9669, 226.8982) -> (1017.0669, 226.9232)
  line L571 (1017.0669, 226.9232) -> (1017.1669, 226.9482)
  line L572 (1017.1669, 226.9482) -> (1017.2669, 226.9732)
  line L573 (1017.2669, 226.9732) -> (1017.3669, 227.0232)
  line L574 (1017.3669, 227.0232) -> (1017.4669, 227.0482)
  line L575 (1017.4669, 227.0482) -> (1017.5669, 227.0982)
  line L576 (1017.5669, 227.0982) -> (1017.6419, 227.1482)
  line L577 (1017.6419, 227.1482) -> (1017.7419, 227.2232)
  line L578 (1017.7419, 227.2232) -> (1017.8169, 227.2982)
  line L579 (1017.8169, 227.2982) -> (1017.8919, 227.3482)
  line L580 (1017.8919, 227.3482) -> (1017.9669, 227.4232)
  line L581 (1017.9669, 227.4232) -> (1018.0419, 227.5232)
  line L582 (1018.0419, 227.5232) -> (1018.092, 227.5982)
  line L583 (1018.092, 227.5982) -> (1018.1419, 227.6982)
  line L584 (1018.1419, 227.6982) -> (1018.1919, 227.7732)
  line L585 (1018.1919, 227.7732) -> (1018.242, 227.8732)
  line L586 (1018.242, 227.8732) -> (1018.267, 227.9731)
  line L587 (1018.267, 227.9731) -> (1018.3169, 228.0732)
  line L588 (1018.3169, 228.0732) -> (1018.3419, 228.1732)
  line L589 (1018.3419, 228.1732) -> (1018.3419, 228.2731)
  line L590 (1018.3419, 228.2731) -> (1018.3669, 228.3982)
  line L591 (1018.3669, 228.3982) -> (1018.3669, 228.4982)
  line L592 (1018.3669, 228.4982) -> (1018.3669, 228.598)
  line L593 (1018.3669, 228.598) -> (1018.3419, 228.698)
  line L594 (1004.467, 240.6984) -> (1004.467, 234.2984)
  line L595 (1004.467, 234.2984) -> (1010.667, 234.2984)
  line L596 (1010.667, 234.2984) -> (1010.667, 240.6984)
  line L597 (1010.667, 240.6984) -> (1004.467, 240.6984)
  line L598 (998.5421, 237.723) -> (998.5421, 237.823)
  line L599 (998.5421, 237.823) -> (998.517, 237.923)
  line L600 (998.517, 237.923) -> (998.467, 238.023)
  line L601 (998.467, 238.023) -> (998.4421, 238.123)
  line L602 (998.4421, 238.123) -> (998.392, 238.223)
  line L603 (998.392, 238.223) -> (998.342, 238.298)
  line L604 (998.342, 238.298) -> (998.292, 238.398)
  line L605 (998.292, 238.398) -> (998.2421, 238.473)
  line L606 (998.2421, 238.473) -> (998.167, 238.573)
  line L607 (998.167, 238.573) -> (998.092, 238.648)
  line L608 (998.092, 238.648) -> (998.017, 238.7231)
  line L609 (998.017, 238.7231) -> (997.942, 238.7731)
  line L610 (997.942, 238.7731) -> (997.8421, 238.8481)
  line L611 (997.8421, 238.8481) -> (997.7671, 238.8981)
  line L612 (997.7671, 238.8981) -> (997.6671, 238.9482)
  line L613 (997.6671, 238.9482) -> (997.5671, 238.9982)
  line L614 (997.5671, 238.9982) -> (997.4671, 239.0233)
  line L615 (997.4671, 239.0233) -> (997.3672, 239.0482)
  line L616 (997.3672, 239.0482) -> (997.2672, 239.0733)
  line L617 (997.2672, 239.0733) -> (997.1672, 239.0984)
  line L618 (997.1672, 239.0984) -> (997.0672, 239.0984)
  line L619 (997.0672, 239.0984) -> (996.9672, 239.0984)
  line L620 (996.9672, 239.0984) -> (996.8671, 239.0984)
  line L621 (996.8671, 239.0984) -> (996.7422, 239.0984)
  line L622 (996.7422, 239.0984) -> (996.6422, 239.0733)
  line L623 (996.6422, 239.0733) -> (996.5422, 239.0483)
  line L624 (996.5422, 239.0483) -> (996.4422, 239.0233)
  line L625 (996.4422, 239.0233) -> (996.3422, 238.9983)
  line L626 (996.3422, 238.9983) -> (996.2422, 238.9483)
  line L627 (996.2422, 238.9483) -> (996.1672, 238.8983)
  line L628 (996.1672, 238.8983) -> (996.0672, 238.8483)
  line L629 (996.0672, 238.8483) -> (995.9921, 238.7733)
  line L630 (995.9921, 238.7733) -> (995.9171, 238.7233)
  line L631 (995.9171, 238.7233) -> (995.8422, 238.6484)
  line L632 (995.8422, 238.6484) -> (995.7672, 238.5734)
  line L633 (995.7672, 238.5734) -> (995.6921, 238.4734)
  line L634 (995.6921, 238.4734) -> (995.6421, 238.3984)
  line L635 (995.6421, 238.3984) -> (995.5671, 238.2984)
  line L636 (995.5671, 238.2984) -> (995.517, 238.2234)
  line L637 (995.517, 238.2234) -> (995.492, 238.1234)
  line L638 (995.492, 238.1234) -> (995.4421, 238.0234)
  line L639 (995.4421, 238.0234) -> (995.417, 237.9234)
  line L640 (995.417, 237.9234) -> (995.3921, 237.8234)
  line L641 (995.3921, 237.8234) -> (995.3671, 237.7234)
  line L642 (995.3671, 237.7234) -> (995.3671, 237.6235)
  line L643 (995.3671, 237.6235) -> (995.3671, 237.4984)
  line L644 (995.3671, 237.4984) -> (995.3671, 237.3985)
  line L645 (995.3671, 237.3985) -> (995.3671, 237.2984)
  line L646 (995.3671, 237.2984) -> (995.3921, 237.1984)
  line L647 (995.3921, 237.1984) -> (995.417, 237.0985)
  line L648 (995.417, 237.0985) -> (995.4421, 236.9984)
  line L649 (995.4421, 236.9984) -> (995.4921, 236.8984)
  line L650 (995.4921, 236.8984) -> (995.5171, 236.7985)
  line L651 (995.5171, 236.7985) -> (995.5671, 236.6984)
  line L652 (995.5671, 236.6984) -> (995.6421, 236.6234)
  line L653 (995.6421, 236.6234) -> (995.692, 236.5484)
  line L654 (995.692, 236.5484) -> (995.7671, 236.4484)
  line L655 (995.7671, 236.4484) -> (995.842, 236.3734)
  line L656 (995.842, 236.3734) -> (995.9169, 236.2983)
  line L657 (995.9169, 236.2983) -> (995.9919, 236.2483)
  line L658 (995.9919, 236.2483) -> (996.0669, 236.1733)
  line L659 (996.0669, 236.1733) -> (996.1669, 236.1233)
  line L660 (996.1669, 236.1233) -> (996.2419, 236.0733)
  line L661 (996.2419, 236.0733) -> (996.3419, 236.0232)
  line L662 (996.3419, 236.0232) -> (996.4419, 235.9982)
  line L663 (996.4419, 235.9982) -> (996.542, 235.9732)
  line L664 (996.542, 235.9732) -> (996.6419, 235.9481)
  line L665 (996.6419, 235.9481) -> (996.7419, 235.9231)
  line L666 (996.7419, 235.9231) -> (996.8668, 235.9231)
  line L667 (996.8668, 235.9231) -> (996.9669, 235.8981)
  line L668 (996.9669, 235.8981) -> (997.0669, 235.9231)
  line L669 (997.0669, 235.9231) -> (997.1669, 235.9231)
  line L670 (997.1669, 235.9231) -> (997.2669, 235.9481)
  line L671 (997.2669, 235.9481) -> (997.3668, 235.9731)
  line L672 (997.3668, 235.9731) -> (997.4668, 235.9981)
  line L673 (997.4668, 235.9981) -> (997.5668, 236.0231)
  line L674 (997.5668, 236.0231) -> (997.6668, 236.0731)
  line L675 (997.6668, 236.0731) -> (997.7668, 236.1231)
  line L676 (997.7668, 236.1231) -> (997.8418, 236.1731)
  line L677 (997.8418, 236.1731) -> (997.9418, 236.2481)
  line L678 (997.9418, 236.2481) -> (998.0168, 236.2981)
  line L679 (998.0168, 236.2981) -> (998.0919, 236.3731)
  line L680 (998.0919, 236.3731) -> (998.1669, 236.448)
  line L681 (998.1669, 236.448) -> (998.242, 236.548)
  line L682 (998.242, 236.548) -> (998.2919, 236.623)
  line L683 (998.2919, 236.623) -> (998.3419, 236.698)
  line L684 (998.3419, 236.698) -> (998.392, 236.798)
  line L685 (998.392, 236.798) -> (998.442, 236.898)
  line L686 (998.442, 236.898) -> (998.467, 236.998)
  line L687 (998.467, 236.998) -> (998.517, 237.098)
  line L688 (998.517, 237.098) -> (998.5421, 237.1979)
  line L689 (998.5421, 237.1979) -> (998.5421, 237.298)
  line L690 (998.5421, 237.298) -> (998.5671, 237.398)
  line L691 (998.5671, 237.398) -> (998.5671, 237.4979)
  line L692 (998.5671, 237.4979) -> (998.5671, 237.623)
  line L693 (998.5671, 237.623) -> (998.5421, 237.723)
  line L694 (983.267, 240.6984) -> (983.267, 234.2984)
  line L695 (983.267, 234.2984) -> (989.467, 234.2984)
  line L696 (989.467, 234.2984) -> (989.467, 240.6984)
  line L697 (989.467, 240.6984) -> (983.267, 240.6984)
  line L698 (987.3418, 228.698) -> (987.3418, 228.798)
  line L699 (987.3418, 228.798) -> (987.3168, 228.898)
  line L700 (987.3168, 228.898) -> (987.2669, 228.998)
  line L701 (987.2669, 228.998) -> (987.2419, 229.098)
  line L702 (987.2419, 229.098) -> (987.1919, 229.1981)
  line L703 (987.1919, 229.1981) -> (987.1419, 229.298)
  line L704 (987.1419, 229.298) -> (987.0919, 229.373)
  line L705 (987.0919, 229.373) -> (987.0419, 229.473)
  line L706 (987.0419, 229.473) -> (986.9669, 229.5481)
  line L707 (986.9669, 229.5481) -> (986.8919, 229.6231)
  line L708 (986.8919, 229.6231) -> (986.8169, 229.6981)
  line L709 (986.8169, 229.6981) -> (986.7419, 229.7481)
  line L710 (986.7419, 229.7481) -> (986.642, 229.8231)
  line L711 (986.642, 229.8231) -> (986.567, 229.8732)
  line L712 (986.567, 229.8732) -> (986.467, 229.9232)
  line L713 (986.467, 229.9232) -> (986.367, 229.9733)
  line L714 (986.367, 229.9733) -> (986.267, 229.9983)
  line L715 (986.267, 229.9983) -> (986.1671, 230.0483)
  line L716 (986.1671, 230.0483) -> (986.0671, 230.0483)
  line L717 (986.0671, 230.0483) -> (985.9671, 230.0734)
  line L718 (985.9671, 230.0734) -> (985.8671, 230.0984)
  line L719 (985.8671, 230.0984) -> (985.7671, 230.0984)
  line L720 (985.7671, 230.0984) -> (985.6671, 230.0984)
  line L721 (985.6671, 230.0984) -> (985.5421, 230.0734)
  line L722 (985.5421, 230.0734) -> (985.4421, 230.0484)
  line L723 (985.4421, 230.0484) -> (985.3421, 230.0484)
  line L724 (985.3421, 230.0484) -> (985.2421, 229.9984)
  line L725 (985.2421, 229.9984) -> (985.1421, 229.9734)
  line L726 (985.1421, 229.9734) -> (985.0421, 229.9234)
  line L727 (985.0421, 229.9234) -> (984.9671, 229.8734)
  line L728 (984.9671, 229.8734) -> (984.8671, 229.8234)
  line L729 (984.8671, 229.8234) -> (984.7921, 229.7484)
  line L730 (984.7921, 229.7484) -> (984.7171, 229.6984)
  line L731 (984.7171, 229.6984) -> (984.6421, 229.6234)
  line L732 (984.6421, 229.6234) -> (984.5671, 229.5484)
  line L733 (984.5671, 229.5484) -> (984.492, 229.4734)
  line L734 (984.492, 229.4734) -> (984.4421, 229.3734)
  line L735 (984.4421, 229.3734) -> (984.3671, 229.2984)
  line L736 (984.3671, 229.2984) -> (984.317, 229.1985)
  line L737 (984.317, 229.1985) -> (984.292, 229.0984)
  line L738 (984.292, 229.0984) -> (984.2421, 228.9984)
  line L739 (984.2421, 228.9984) -> (984.2171, 228.8985)
  line L740 (984.2171, 228.8985) -> (984.192, 228.7984)
  line L741 (984.192, 228.7984) -> (984.167, 228.6984)
  line L742 (984.167, 228.6984) -> (984.167, 228.5984)
  line L743 (984.167, 228.5984) -> (984.167, 228.4984)
  line L744 (984.167, 228.4984) -> (984.167, 228.3984)
  line L745 (984.167, 228.3984) -> (984.167, 228.2734)
  line L746 (984.167, 228.2734) -> (984.192, 228.1735)
  line L747 (984.192, 228.1735) -> (984.2171, 228.0734)
  line L748 (984.2171, 228.0734) -> (984.2421, 227.9734)
  line L749 (984.2421, 227.9734) -> (984.292, 227.8735)
  line L750 (984.292, 227.8735) -> (984.317, 227.7734)
  line L751 (984.317, 227.7734) -> (984.3671, 227.6985)
  line L752 (984.3671, 227.6985) -> (984.4421, 227.5985)
  line L753 (984.4421, 227.5985) -> (984.4921, 227.5235)
  line L754 (984.4921, 227.5235) -> (984.5671, 227.4235)
  line L755 (984.5671, 227.4235) -> (984.6421, 227.3484)
  line L756 (984.6421, 227.3484) -> (984.7171, 227.2984)
  line L757 (984.7171, 227.2984) -> (984.7921, 227.2234)
  line L758 (984.7921, 227.2234) -> (984.867, 227.1483)
  line L759 (984.867, 227.1483) -> (984.967, 227.0983)
  line L760 (984.967, 227.0983) -> (985.042, 227.0483)
  line L761 (985.042, 227.0483) -> (985.1419, 227.0233)
  line L762 (985.1419, 227.0233) -> (985.2419, 226.9732)
  line L763 (985.2419, 226.9732) -> (985.3419, 226.9482)
  line L764 (985.3419, 226.9482) -> (985.4419, 226.9231)
  line L765 (985.4419, 226.9231) -> (985.542, 226.8981)
  line L766 (985.542, 226.8981) -> (985.6669, 226.8981)
  line L767 (985.6669, 226.8981) -> (985.7669, 226.8981)
  line L768 (985.7669, 226.8981) -> (985.8669, 226.8981)
  line L769 (985.8669, 226.8981) -> (985.9669, 226.8981)
  line L770 (985.9669, 226.8981) -> (986.0669, 226.9231)
  line L771 (986.0669, 226.9231) -> (986.1669, 226.9481)
  line L772 (986.1669, 226.9481) -> (986.2669, 226.9731)
  line L773 (986.2669, 226.9731) -> (986.3669, 227.0231)
  line L774 (986.3669, 227.0231) -> (986.4669, 227.0481)
  line L775 (986.4669, 227.0481) -> (986.5669, 227.0981)
  line L776 (986.5669, 227.0981) -> (986.6419, 227.1481)
  line L777 (986.6419, 227.1481) -> (986.7419, 227.2231)
  line L778 (986.7419, 227.2231) -> (986.8169, 227.2981)
  line L779 (986.8169, 227.2981) -> (986.8919, 227.3481)
  line L780 (986.8919, 227.3481) -> (986.9668, 227.4231)
  line L781 (986.9668, 227.4231) -> (987.0419, 227.5231)
  line L782 (987.0419, 227.5231) -> (987.0919, 227.5981)
  line L783 (987.0919, 227.5981) -> (987.1419, 227.6981)
  line L784 (987.1419, 227.6981) -> (987.1919, 227.7731)
  line L785 (987.1919, 227.7731) -> (987.242, 227.8731)
  line L786 (987.242, 227.8731) -> (987.267, 227.9731)
  line L787 (987.267, 227.9731) -> (987.3169, 228.0731)
  line L788 (987.3169, 228.0731) -> (987.3419, 228.1731)
  line L789 (987.3419, 228.1731) -> (987.3419, 228.2731)
  line L790 (987.3419, 228.2731) -> (987.3669, 228.3981)
  line L791 (987.3669, 228.3981) -> (987.3669, 228.4981)
  line L792 (987.3669, 228.4981) -> (987.3669, 228.598)
  line L793 (987.3669, 228.598) -> (987.3418, 228.698)
  line L794 (967.1921, 231.9734) -> (966.942, 232.5734)
  line L795 (966.942, 232.5734) -> (966.5421, 233.0984)
  line L796 (966.5421, 233.0984) -> (966.017, 233.4984)
  line L797 (966.017, 233.4984) -> (965.4171, 233.7484)
  line L798 (965.4171, 233.7484) -> (964.7671, 233.8234)
  line L799 (964.7671, 233.8234) -> (964.1171, 233.7484)
  line L800 (964.1171, 233.7484) -> (963.492, 233.4984)
  line L801 (963.492, 233.4984) -> (962.9671, 233.0984)
  line L802 (962.9671, 233.0984) -> (962.5671, 232.5734)
  line L803 (962.5671, 232.5734) -> (962.3171, 231.9734)
  line L804 (962.3171, 231.9734) -> (962.242, 231.2984)
  line L805 (962.242, 231.2984) -> (962.3171, 230.6484)
  line L806 (962.3171, 230.6484) -> (962.5671, 230.0484)
  line L807 (962.5671, 230.0484) -> (962.9671, 229.5234)
  line L808 (962.9671, 229.5234) -> (963.492, 229.1235)
  line L809 (963.492, 229.1235) -> (964.1171, 228.8735)
  line L810 (964.1171, 228.8735) -> (964.7671, 228.7986)
  line L811 (964.7671, 228.7986) -> (965.4171, 228.8736)
  line L812 (965.4171, 228.8736) -> (966.017, 229.1236)
  line L813 (966.017, 229.1236) -> (966.5421, 229.5236)
  line L814 (966.5421, 229.5236) -> (966.9421, 230.0486)
  line L815 (966.9421, 230.0486) -> (967.1921, 230.6486)
  line L816 (967.1921, 230.6486) -> (967.267, 231.2986)
  line L817 (967.267, 231.2986) -> (967.1921, 231.9734)
  line L818 (1021.9429, 238.0232) -> (1021.9178, 238.3482)
  line L819 (1021.9178, 238.3482) -> (1021.8678, 238.6732)
  line L820 (1021.8678, 238.6732) -> (1021.7928, 238.9732)
  line L821 (1021.7928, 238.9732) -> (1021.6927, 239.2982)
  line L822 (1021.6927, 239.2982) -> (1021.5928, 239.5982)
  line L823 (1021.5928, 239.5982) -> (1021.4429, 239.8983)
  line L824 (1021.4429, 239.8983) -> (1021.2928, 240.1983)
  line L825 (1021.2928, 240.1983) -> (1021.1178, 240.4732)
  line L826 (1021.1178, 240.4732) -> (1020.9178, 240.7232)
  line L827 (1020.9178, 240.7232) -> (1020.7178, 240.9982)
  line L828 (1020.7178, 240.9982) -> (1020.4929, 241.2233)
  line L829 (1020.4929, 241.2233) -> (1020.2679, 241.4483)
  line L830 (1020.2679, 241.4483) -> (1020.018, 241.6484)
  line L831 (1020.018, 241.6484) -> (1019.7431, 241.8485)
  line L832 (1019.7431, 241.8485) -> (1019.4681, 242.0235)
  line L833 (1019.4681, 242.0235) -> (1019.1682, 242.1737)
  line L834 (1019.1682, 242.1737) -> (1018.8681, 242.2987)
  line L835 (1018.8681, 242.2987) -> (1018.5682, 242.4237)
  line L836 (1018.5682, 242.4237) -> (1018.2682, 242.5238)
  line L837 (1018.2682, 242.5238) -> (1017.9432, 242.5989)
  line L838 (1017.9432, 242.5989) -> (1017.6182, 242.6489)
  line L839 (1017.6182, 242.6489) -> (1017.2933, 242.6739)
  line L840 (1017.2933, 242.6739) -> (1016.9682, 242.699)
  line L841 (1016.9682, 242.699) -> (949.7668, 242.699)
  line L842 (949.7668, 242.699) -> (949.7668, 182.6984)
  line L843 (949.7668, 182.6984) -> (1016.9668, 182.6984)
  line L844 (1016.9668, 182.6984) -> (1017.2919, 182.6984)
  line L845 (1017.2919, 182.6984) -> (1017.6168, 182.7234)
  line L846 (1017.6168, 182.7234) -> (1017.9418, 182.7984)
  line L847 (1017.9418, 182.7984) -> (1018.2668, 182.8734)